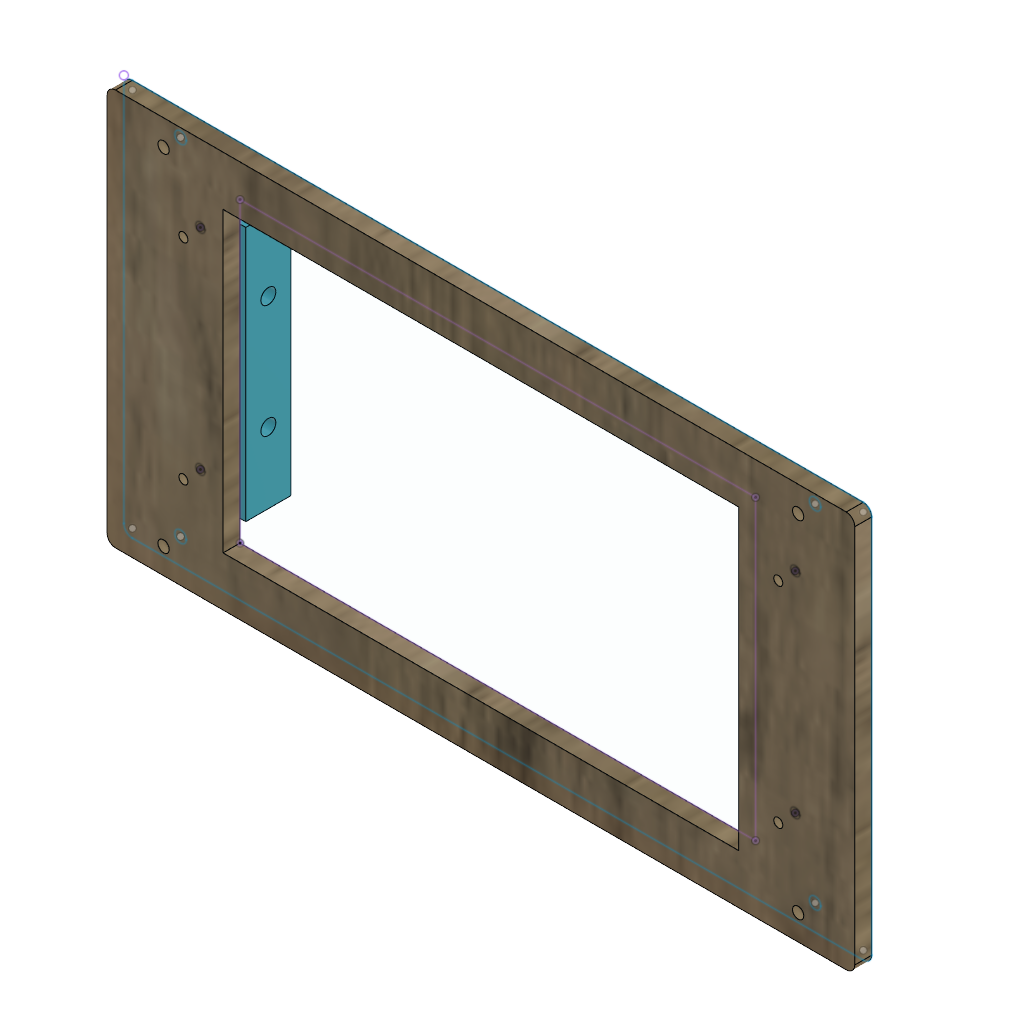
esgoo_stereo_mount (Autodesk Fusion 360 design; units mm, degrees)
part number: 2026-10-01-11-48-25-005
Autodesk Fusion 360 part; units mm, degrees
ref_plane "WorkPlane1" through (43, 0, 0) normal (1, 0, 0) x (0, 1, 0)
ref_plane "WorkPlane2" through (132, 0, 0) normal (1, 0, 0) x (0, 1, 0)
sketch "dimensions" plane through (0, 0, 0) normal (0, 1, 0) x (1, 0, 0)
  line L0 (0, 0) -> (264, 0)
  line L1 (264, 0) -> (264, -140)
  line L2 (264, -140) -> (0, -140)
  line L3 (0, -140) -> (0, 0)
  line L4 (132, -140) -> (132, 0) construction
  line L5 (264, -70) -> (0, -70) construction
  line L6 (257.4125, -120.8) -> (6.5875, -120.8) construction
  line L7 (6.5875, -120.8) -> (6.5875, -19.2) construction
  line L8 (6.5875, -19.2) -> (257.4125, -19.2) construction
  line L9 (257.4125, -19.2) -> (257.4125, -120.8) construction
  line L10 (257.4125, -120.8) -> (6.5875, -19.2) construction
  line L11 (6.5875, -120.8) -> (257.4125, -19.2) construction
  line L12 (41, -122.5) -> (223, -122.5)
  line L13 (223, -122.5) -> (223, -17.5)
  line L14 (223, -17.5) -> (41, -17.5)
  line L15 (41, -17.5) -> (41, -122.5)
  line L16 (41, -122.5) -> (223, -17.5) construction
  line L17 (223, -122.5) -> (41, -17.5) construction
  line L18 (43, -140) -> (43, 0) construction
  line L19 (221, -140) -> (221, 0) construction
  line L20 (43, -33) -> (27, -33) construction
  line L21 (43, -107) -> (27, -107) construction
  line L22 (221, -107) -> (237, -107) construction
  line L23 (221, -33) -> (237, -33) construction
  circle A0 centre (27, -107) radius 1.4
  circle A1 centre (27, -33) radius 1.4
  circle A2 centre (237, -107) radius 1.4
  circle A3 centre (237, -33) radius 1.4
  point P0 (132, -70)
  point P1 (132, -70)
  point P2 (132, -70)
  point P3 (43, -70)
  point P4 (221, -70)
  dimension "d1" = 264
  dimension "d2" = 140
  dimension "d3" = 250.825
  dimension "d4" = 101.6
  dimension "d5" = 182
  dimension "d6" = 105
  dimension "d7" = 43
  dimension "d8" = 43
  dimension "d23" = 16
  dimension "d24" = 16
  dimension "d25" = 37
  dimension "d26" = 37
  dimension "d27" = 16
  dimension "d28" = 16
  dimension "d29" = 37
  dimension "d30" = 37
  dimension "d31" = 2.8
  dimension "d32" = 2.8
  dimension "d33" = 2.8
  dimension "d34" = 2.8
  dimension "d58" = 132
  constraint horizontal L0
  constraint vertical L1
  constraint horizontal L2
  constraint vertical L3
  constraint coincident L0.start L3.end
  constraint midpoint L2 L4.start
  constraint midpoint L0 L4.end
  constraint midpoint L1 L5.start
  constraint midpoint L3 L5.end
  constraint midpoint L4 P2
  constraint horizontal L6
  constraint perpendicular L6 L7
  constraint parallel L6 L8
  constraint parallel L7 L9
  constraint coincident L10 P2
  constraint coincident L11 P2
  constraint coincident P2 P1
  constraint horizontal L12
  constraint perpendicular L12 L13
  constraint parallel L12 L14
  constraint parallel L13 L15
  constraint coincident L16 P2
  constraint coincident L17 P2
  constraint coincident L2 L18.start
  constraint coincident L0 L18.end
  constraint perpendicular L0 L18
  constraint coincident L2 L19.start
  constraint coincident L0 L19.end
  constraint perpendicular L0 L19
  constraint midpoint L18 P3
  constraint coincident L18 L20.start
  constraint perpendicular L15 L20
  constraint coincident L18 L21.start
  constraint perpendicular L15 L21
  constraint midpoint L19 P4
  constraint coincident L19 L22.start
  constraint perpendicular L13 L22
  constraint coincident L19 L23.start
  constraint perpendicular L13 L23
  constraint coincident L21.end A0.centre
  constraint coincident L20.end A1.centre
  constraint coincident L22.end A2.centre
  constraint coincident L23.end A3.centre
  measures "d1" distance of L0.start L0.end
  measures "d2" distance of L0.start L2.end
  measures "d3" distance of L7.end L8.end
  measures "d4" distance of L6.end L7.end
  measures "d5" distance of L13.end L14.end
  measures "d6" distance of L12.end L13.end
  measures "d7" distance of L2.end L18.start
  measures "d8" distance of L1.end L19.start
  measures "d23" distance of L20.start L20.end
  measures "d24" distance of L21.start L21.end
  measures "d25" distance of P3 L21.start
  measures "d26" distance of P3 L20.start
  measures "d27" distance of L22.start L22.end
  measures "d28" distance of L23.start L23.end
  measures "d29" distance of P4 L23.start
  measures "d30" distance of P4 L22.start
  measures "d31" diameter of A0
  measures "d32" diameter of A1
  measures "d33" diameter of A2
  measures "d34" diameter of A3
  measures "d58" distance of L0.start L4.end
sketch "left-bracket" plane through (43, 0, 0) normal (1, 0, 0) x (0, 1, 0)
  line L0 (0, 70) -> (8, 70) construction
  line L1 (8, 70) -> (8, 90) construction
  line L2 (8, 70) -> (8, 50) construction
  circle A0 centre (8, 90) radius 2.65
  circle A1 centre (8, 50) radius 2.65
  line L3 (5.6906, 94) -> (3.3812, 90) construction
  line L4 (3.3812, 90) -> (5.6906, 86) construction
  line L5 (5.6906, 86) -> (10.3094, 86) construction
  line L6 (10.3094, 86) -> (12.6188, 90) construction
  line L7 (12.6188, 90) -> (10.3094, 94) construction
  line L8 (10.3094, 94) -> (5.6906, 94) construction
  line L9 (5.6906, 54) -> (3.3812, 50) construction
  line L10 (3.3812, 50) -> (5.6906, 46) construction
  line L11 (5.6906, 46) -> (10.3094, 46) construction
  line L12 (10.3094, 46) -> (12.6188, 50) construction
  line L13 (12.6188, 50) -> (10.3094, 54) construction
  line L14 (10.3094, 54) -> (5.6906, 54) construction
  line L15 (0, 70) -> (0, 25) construction
  line L16 (0, 25) -> (16, 25)
  line L17 (16, 25) -> (16, 115)
  line L18 (16, 115) -> (0, 115)
  line L19 (0, 115) -> (0, 25)
  line L20 (16, 99) -> (0, 99)
  line L21 (16, 41) -> (0, 41)
  point P0 (0, 70)
  point P1 (8, 90)
  point P2 (8, 50)
  dimension "d11" = 8
  dimension "d12" = 20
  dimension "d13" = 20
  dimension "d14" = 5.3
  dimension "d15" = 5.3
  dimension "d16" = 4
  dimension "d17" = 4
  dimension "d18" = 45
  dimension "d19" = 16
  dimension "d20" = 90
  dimension "d21" = 16
  dimension "d22" = 16
  constraint coincident P0 L0.start
  constraint horizontal L0
  constraint perpendicular L0 L1
  constraint perpendicular L0 L2
  constraint coincident P1 L1.end
  constraint coincident P2 L2.end
  constraint perpendicular L0 L15
  constraint horizontal L16
  constraint vertical L17
  constraint horizontal L18
  constraint vertical L19
  constraint coincident L17 L20.start
  constraint coincident L19 L20.end
  constraint perpendicular L19 L20
  constraint coincident L17 L21.start
  constraint coincident L19 L21.end
  constraint horizontal L21
  measures "d11" distance of P0 L0.end
  measures "d12" distance of L0.end P1
  measures "d13" distance of L0.end P2
  measures "d14" diameter of A0
  measures "d15" diameter of A1
  measures "d16" distance of P1 L8
  measures "d17" distance of P2 L14
  measures "d18" distance of P0 L15.end
  measures "d19" distance of L15.end L16.end
  measures "d20" distance of L15.end L18.end
  measures "d21" distance of L17.end L20.start
  measures "d22" distance of L16.end L21.start
sketch "esgoo_wood" plane through (0, 0, 0) normal (0, 1, 0) x (1, 0, 0)
  line L0 (3, 0) -> (261, 0)
  line L1 (264, -3) -> (264, -137)
  line L2 (0, -137) -> (0, -3)
  line L3 (261, -140) -> (3, -140)
  line L4 (41, -17.5) -> (41, -122.5)
  line L5 (41, -122.5) -> (223, -122.5)
  line L6 (223, -17.5) -> (41, -17.5)
  line L7 (223, -122.5) -> (223, -17.5)
  circle A0 centre (27, -107) radius 1.6
  circle A1 centre (27, -33) radius 1.6
  circle A2 centre (237, -107) radius 1.6
  circle A3 centre (237, -33) radius 1.6
  circle A4 centre (20, -131) radius 2
  circle A5 centre (244, -131) radius 2
  circle A6 centre (244, -9) radius 2
  circle A7 centre (20, -9) radius 2
  arc A8 (0, -137) -> (3, -140) centre (3, -137) ccw
  arc A9 (261, -140) -> (264, -137) centre (261, -137) ccw
  arc A10 (264, -3) -> (261, 0) centre (261, -3) ccw
  arc A11 (3, 0) -> (0, -3) centre (3, -3) ccw
  point P0 (27, -107)
  point P1 (27, -33)
  point P2 (237, -33)
  point P3 (237, -107)
  point P4 (0, -140)
  dimension "d35" = 3.2
  dimension "d36" = 3.2
  dimension "d37" = 3.2
  dimension "d38" = 3.2
  dimension "d39" = 4
  dimension "d40" = 20
  dimension "d41" = 9
  dimension "d42" = 4
  dimension "d43" = 4
  dimension "d44" = 4
  dimension "d45" = 20
  dimension "d46" = 9
  dimension "d47" = 20
  dimension "d48" = 9
  dimension "d49" = 20
  dimension "d50" = 9
  dimension "d51" = 3
  constraint coincident P0 A0.centre
  constraint coincident P1 A1.centre
  constraint coincident P3 A2.centre
  constraint coincident P2 A3.centre
  constraint tangent L2 A8
  constraint tangent L3 A8
  constraint tangent L3 A9
  constraint tangent L1 A9
  constraint equal A8 A9
  constraint tangent L1 A10
  constraint tangent L0 A10
  constraint equal A8 A10
  constraint tangent L0 A11
  constraint tangent L2 A11
  constraint equal A8 A11
  measures "d35" diameter of A0
  measures "d36" diameter of A1
  measures "d37" diameter of A2
  measures "d38" diameter of A3
  measures "d39" diameter of A4
  measures "d40" distance of L2 A4.centre
  measures "d41" vertical distance of A4.centre P4
  measures "d42" diameter of A5
  measures "d43" diameter of A6
  measures "d44" diameter of A7
  measures "d45" distance of L2 A7.centre
  measures "d46" distance of L0 A7.centre
  measures "d47" distance of L1 A5.centre
  measures "d48" distance of L3 A5.centre
  measures "d49" distance of L1 A6.centre
  measures "d50" distance of L0 A6.centre
  measures "d51" radius of A8
extrude "Extrude1" add sketch "left-bracket" against normal blind 5 contours L17 L19 L20 L21 makes body 1
extrude "Extrude2" add sketch "left-bracket" against normal blind 26 contours L16 L17 L19 L21 | L17 L18 L19 L20 bodies 1
extrude "Extrude3" cut sketch "dimensions" along normal blind 16 contours A0 | A1 bodies 1
mirror "Mirror1" about plane through (132, 0, 0) normal (1, 0, 0) of bodies 1 makes body 2
extrude "Extrude4" add sketch "esgoo_wood" against normal blind 6 separate body makes body 3
equation "d3 = 9 7/8\""
equation "d4 = 4\""
equation "d25 = 45 mm - 8 mm"
equation "d26 = 45 mm - 8 mm"
equation "d29 = 45 mm - 8 mm"
equation "d30 = 45 mm - 8 mm"
